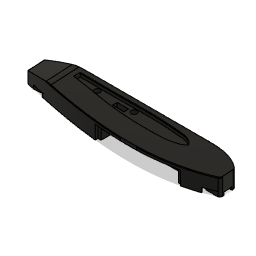
Rumpffräsung (Autodesk Fusion 360 archive; units mm, degrees)
design "Victor900_Rumpf_L"
Autodesk Fusion 360 part; units mm, degrees
(part 1 of 2)
sketch "Skizze1" plane through (0, 0, 0) normal (0, 1, 0) x (1, 0, 0)
  line L0 (-130, 18) -> (210, 18)
  line L1 (210, 18) -> (210, -52)
  line L2 (210, -52) -> (-130, -52)
  line L3 (-130, -52) -> (-130, 18)
  dimension "d132" = 70
  dimension "d133" = 130
  dimension "d134" = 18
  dimension "d135" = 340
  constraint horizontal L0
  constraint vertical L1
  constraint horizontal L2
  constraint vertical L3
  measures "d132" distance of L0.start L2.end
  measures "d133" distance of origin L3
  measures "d134" distance of origin L0
  measures "d135" distance of L1.end L2.end
extrude "Extrusion1" add sketch "Skizze1" along normal blind 5 and the other way blind 25
sketch "Skizze2" plane through (0, 5, 0) normal (0, 1, 0) x (-1, 0, 0)
  line L0 (130, 52) -> (-210, 52)
  line L1 (-210, 52) -> (-210, -18)
  line L2 (-210, -18) -> (130, -18)
  line L3 (130, -18) -> (130, 52)
  spline S0 degree 5 poles (-210, 26) (-205.2364, 28.1616) (-195.5185, 32.2752) (-180.3701, 37.8161) (-159.0102, 43.925) (-130.2557, 49.2993) (-99.3092, 52.2606) (-66.073, 52.7014) (-30.619, 50.7009) (6.8654, 46.4652) (46.175, 40.2203) (78.9412, 33.773) (104.2065, 28.1772) (121.3518, 24.1145) (130, 22) knots 0 0 0 0 0 0 0.1 0.2 0.3 0.4 0.5 0.6 0.7 0.8 0.9 1 1 1 1 1 1
  spline S1 degree 5 poles (-210, 2) (-208.6315, 0.7563) (-205.7512, -1.6794) (-201.0016, -5.1784) (-193.7504, -9.5129) (-182.4072, -14.1098) (-170.3603, -16.7165) (-158.8134, -17.7665) (-149.8205, -18) (-145, -18) knots 0 0 0 0 0 0 0.2 0.4 0.6 0.8 1 1 1 1 1 1
  line L4 (-155, -18) -> (-135, -18)
  spline S2 degree 5 poles (130, -8) (127.9223, -8.6218) (123.6828, -9.8397) (117.0718, -11.5892) (107.7186, -13.7564) (94.6903, -16.0549) (82.5244, -17.3582) (71.9269, -17.8833) (64.1023, -18) (60, -18) knots 0 0 0 0 0 0 0.2 0.4 0.6 0.8 1 1 1 1 1 1
  line L5 (70, -18) -> (50, -18)
  line L6 (-210, 26) -> (-207.3088, -18)
  point P0 (-90, 52)
  dimension "d140" = 120
  dimension "d143" = 20
  dimension "d145" = 24
  dimension "d146" = 65
  dimension "d147" = 30
  dimension "d148" = 20
  dimension "d149" = 70
  dimension "d161" = 3.5
  dimension "d351" = 20
  dimension "d352" = 10
  constraint coincident L1 S0.start
  constraint coincident L0 P0
  constraint coincident L3 S0.end
  constraint coincident L1 S1.start
  constraint coincident L2 S1.end
  constraint midpoint S1.end L4
  constraint collinear L2 L4
  constraint coincident L3 S2.start
  constraint coincident L2 S2.end
  constraint midpoint S2.end L5
  constraint collinear L2 L5
  constraint coincident L2 L6.end
  measures "d140" distance of L1 P0
  measures "d143" distance of L4.start L4.end
  measures "d145" distance of S0.start S1.start
  measures "d146" distance of L1 S1.end
  measures "d147" distance of S0.end S2.start
  measures "d148" distance of L5.start L5.end
  measures "d149" distance of L3 S2.end
  measures "d161" angle of L1 L6
  measures "d351" distance of L1.end S1.start
  measures "d352" distance of L2.end S2.start
extrude "Extrusion2" cut sketch "Skizze2" against normal blind 40 contours L0 L3 S0 | L0 L1 S0 | L2 L3 S2 L5 | L1 S1 L6 | L1 L2 S1 L6 | L2 S1 L4 L6
sketch "Skizze3" plane through (0, 5, 0) normal (0, 1, 0) x (-1, 0, 0)
  spline S0 degree 5 poles (-208.4486, 0.6348) (-207.3338, -0.3155) (-204.6874, -2.4507) (-200.1926, -5.6566) (-193.2477, -9.7166) (-182.4072, -14.1098) (-170.3603, -16.7165) (-158.8134, -17.7665) (-149.8205, -18) (-145, -18) knots 0.044317 0.044317 0.044317 0.044317 0.044317 0.044317 0.2 0.4 0.6 0.8 1 1 1 1 1 1
  line L0 (-145, -18) -> (60, -18)
  spline S1 degree 5 poles (60, -18) (64.1023, -18) (71.9269, -17.8833) (82.5244, -17.3582) (94.6903, -16.0549) (107.7186, -13.7564) (117.0718, -11.5892) (123.6828, -9.8397) (127.9223, -8.6218) (130, -8) knots -1 -1 -1 -1 -1 -1 -0.8 -0.6 -0.4 -0.2 0 0 0 0 0 0
  line L1 (130, -8) -> (130, 22)
  spline S2 degree 5 poles (130, 22) (121.3518, 24.1145) (104.2065, 28.1772) (78.9412, 33.773) (46.175, 40.2203) (7.677, 46.3363) (-21.5732, 49.6777) (-42.4683, 51.2272) (-55.7647, 51.8176) (-61.9632, 52) knots -1 -1 -1 -1 -1 -1 -0.9 -0.8 -0.7 -0.6 -0.510324 -0.510324 -0.510324 -0.510324 -0.510324 -0.510324
  line L2 (-61.9632, 52) -> (-90, 52)
  line L3 (130, -8) -> (128.4074, 22.3885)
  line L4 (129.2037, 7.1943) -> (-168.7369, -8.4202) construction
  line L5 (-210, 26) -> (-208.4486, 0.6348)
  spline S3 degree 5 poles (-90, 52) (-91.7641, 51.9445) (-100.03, 51.6408) (-114.4799, 50.739) (-134.4555, 48.5144) (-159.0102, 43.925) (-180.3701, 37.8161) (-195.5185, 32.2752) (-205.2364, 28.1616) (-210, 26) knots -0.426972 -0.426972 -0.426972 -0.426972 -0.426972 -0.426972 -0.4 -0.3 -0.2 -0.1 0 0 0 0 0 0
  dimension "d154" = 3
  constraint coincident S1.end L1.start
  constraint coincident S2 L3.end
  constraint midpoint L3 L4.start
  constraint perpendicular L3 L4
  measures "d154" angle of L1 L3
extrude "Extrusion3" cut sketch "Skizze3" against normal blind 47 contours L1 S2 L3
ref_plane "Arbeitsebene1" through (40, 0, 17) normal (0, 1, 0) x (0, 0, 1)
sketch "Skizze4" plane through (27.5, 0, 3) normal (0, 1, 0) x (1, 0, 0)
  line L0 (-97.7103, 1.804) -> (-97.7103, 13.2279)
  spline S0 degree 5 poles (-97.7103, 13.2279) (-96.5236, 13.2308) (-93.9185, 13.2352) (-90.1894, 13.2341) (-85.749, 13.2174) (-80.8951, 13.1754) (-76.1251, 13.1176) (-71.0655, 13.0567) (-65.2033, 13.0032) (-58.2308, 12.9668) (-50.1822, 12.9539) (-41.3331, 12.9683) (-32.096, 13.0103) (-22.9177, 13.0771) (-14.1775, 13.1622) (-6.0829, 13.255) (1.4285, 13.3413) (8.5923, 13.4029) (15.7306, 13.4191) (23.1596, 13.3663) (31.1056, 13.2202) (39.6032, 12.953) (48.4974, 12.5463) (57.5071, 11.9937) (66.2205, 11.3341) (74.2213, 10.6113) (80.9203, 10.0066) (86.1005, 9.5493) (90.5962, 8.6856) (95.1878, 6.918) (99.7425, 4.2895) (102.7176, 1.9586) (104.0892, 0.3889) (104.5631, -0.5029) (104.6892, -0.8472) knots -0.850912 -0.850912 -0.850912 -0.850912 -0.850912 -0.850912 -0.828571 -0.8 -0.771429 -0.742857 -0.714286 -0.685714 -0.657143 -0.628571 -0.6 -0.571429 -0.542857 -0.514286 -0.485714 -0.457143 -0.428571 -0.4 -0.371429 -0.342857 -0.314286 -0.285714 -0.257143 -0.228571 -0.2 -0.171429 -0.142857 -0.114286 -0.085714 -0.057143 -0.028571 -0.009156 -0.009156 -0.009156 -0.009156 -0.009156 -0.009156
  spline S1 degree 3 poles (104.6892, -0.8472) (104.7839, -1.1058) (104.8386, -1.3762) (104.8386, -1.6214) (104.8386, -2.5356) (104.213, -3.5125) (103.0553, -4.509) (101.9361, -5.4725) (100.3269, -6.4501) (98.4058, -7.3673) (96.5485, -8.2542) (94.4054, -9.0815) (92.1316, -9.8016) (89.9332, -10.4978) (87.6126, -11.0945) (85.2619, -11.5861) (82.9892, -12.0615) (80.6879, -12.4397) (78.4044, -12.7378) (74.0423, -13.3073) (69.7631, -13.5879) (65.6078, -13.7673) (61.7251, -13.9348) (57.9384, -14.0206) (54.1004, -14.0826) (50.5143, -14.1405) (46.8739, -14.1725) (43.0512, -14.1644) (39.4793, -14.1567) (35.7425, -14.1108) (31.8309, -14.012) (28.176, -13.9197) (24.3726, -13.7815) (20.5153, -13.6027) (16.9111, -13.4356) (13.2643, -13.2337) (9.6785, -13.0077) (6.328, -12.7966) (3.0333, -12.5647) (-0.1432, -12.3189) (-3.1112, -12.0892) (-5.9746, -11.8475) (-8.7301, -11.5932) (-11.3049, -11.3556) (-13.7868, -11.1067) (-16.2144, -10.8408) (-18.4827, -10.5922) (-20.7048, -10.3285) (-22.929, -10.0433) (-27.0353, -9.5168) (-31.1588, -8.9145) (-35.5916, -8.2103) (-39.4497, -7.5975) (-43.5436, -6.9077) (-47.9372, -6.155) (-51.7612, -5.4998) (-55.8084, -4.7979) (-60.059, -4.0715) (-63.7585, -3.4393) (-67.6104, -2.7889) (-71.5828, -2.1377) (-78.4142, -1.0179) (-85.5958, 0.1013) (-92.9594, 1.1447) (-94.5348, 1.368) (-96.1189, 1.5879) (-97.7103, 1.804) knots 0 0 0 0 0.00882694 0.00882694 0.00882694 0.04173953 0.04173953 0.04173953 0.07355923 0.07355923 0.07355923 0.10432234 0.10432234 0.10432234 0.13406394 0.13406394 0.13406394 0.16281794 0.16281794 0.16281794 0.21774546 0.21774546 0.21774546 0.26906918 0.26906918 0.26906918 0.31702555 0.31702555 0.31702555 0.3618355 0.3618355 0.3618355 0.40370548 0.40370548 0.40370548 0.44282836 0.44282836 0.44282836 0.47938439 0.47938439 0.47938439 0.51354198 0.51354198 0.51354198 0.54545849 0.54545849 0.54545849 0.57528096 0.57528096 0.57528096 0.63034008 0.63034008 0.63034008 0.67826152 0.67826152 0.67826152 0.7199706 0.7199706 0.7199706 0.75627265 0.75627265 0.75627265 0.81870207 0.81870207 0.81870207 0.8320585 0.8320585 0.8320585 0.8320585
extrude "Extrusion4" cut sketch "Skizze4" along normal blind 30
fillet "Abrundung2" radius 5 2 edges at (210, -10, 26) (208.4486, -10, 0.6348)
sketch "Skizze6" plane through (0, -25, 0) normal (0, -1, 0) x (1, 0, 0)
  spline S0 degree 3 poles (208.5813, 2.8044) (208.5416, 2.1546) (208.3753, 1.5187) (207.9292, 0.5965) (207.7295, 0.2796) (207.2633, -0.3037) (206.9983, -0.5683) (206.7063, -0.8009) knots 0 0 0 0 0.195322 0.195322 0.307328 0.307328 0.419333 0.419333 0.419333 0.419333
  line L0 (208.5813, 2.8044) -> (209.7883, 22.5389)
  line L1 (90, 52) -> (61.9632, 52)
  spline S1 degree 3 poles (61.9632, 52) (31.8484, 51.1138) (0.7584, 47.5087) (-61.8469, 37.484) (-95.8238, 30.3193) (-128.4074, 22.3885) knots 0 0 0 0 9.038353 9.038353 19.164916 19.164916 19.164916 19.164916
  line L2 (-128.4074, 22.3885) -> (-130, -8)
  spline S2 degree 3 poles (-130, -8) (-122.2961, -10.3057) (-112.1158, -12.9457) (-88.0124, -17.0435) (-75.2267, -18) (-60, -18) knots 0 0 0 0 2.412467 2.412467 5.223942 5.223942 5.223942 5.223942
  line L3 (-60, -18) -> (145, -18)
  spline S3 degree 3 poles (145, -18) (162.314, -18) (175.3428, -16.1927) (195.2364, -8.9464) (201.9978, -4.5522) (206.7063, -0.8009) knots 0 0 0 0 5.194191 5.194191 9.349234 9.349234 9.349234 9.349234
  line L4 (209.6335, 20.0079) -> (199.6522, 20.6184)
  line L5 (199.6522, 20.6184) -> (198.7547, 5.9458)
  line L6 (198.7547, 5.9458) -> (208.7361, 5.3354)
  line L7 (209.1848, 12.6716) -> (199.2035, 13.2821) construction
  line L8 (199.6522, 20.6184) -> (199.7987, 23.0139)
  line L9 (199.7987, 23.0139) -> (187.8211, 23.7465)
  line L10 (187.8211, 23.7465) -> (186.6306, 4.2829)
  line L11 (186.6306, 4.2829) -> (198.6082, 3.5503)
  line L12 (198.6082, 3.5503) -> (198.7547, 5.9458)
  line L13 (187.2258, 14.0147) -> (199.2035, 13.2821) construction
  spline S4 degree 3 poles (206.8011, 27.4252) (207.3976, 27.1643) (207.9375, 26.7894) (208.8431, 25.8537) (209.2002, 25.3019) (209.5778, 24.3557) (209.676, 24.0003) (209.7927, 23.2742) (209.8108, 22.9059) (209.7883, 22.5389) knots 0 0 0 0 0.195322 0.195322 0.390644 0.390644 0.500949 0.500949 0.611253 0.611253 0.611253 0.611253
  spline S5 degree 3 poles (206.8011, 27.4252) (190.0948, 34.7315) (172.6088, 40.2679) (133.4369, 48.918) (111.8704, 51.3122) (90, 52) knots 0.350203 0.350203 0.350203 0.350203 5.82041 5.82041 12.339895 12.339895 12.339895 12.339895
  dimension "d164" = 14.7
  dimension "d165" = 10
  dimension "d166" = 19.5
  dimension "d168" = 12
  constraint coincident L0 L4.start
  constraint perpendicular L0 L4
  constraint perpendicular L4 L5
  constraint coincident L0 L6.end
  constraint perpendicular L0 L6
  constraint midpoint L0 L7.start
  constraint midpoint L5 L7.end
  constraint perpendicular L5 L7
  constraint perpendicular L4 L8
  constraint perpendicular L8 L9
  constraint perpendicular L10 L11
  constraint perpendicular L6 L12
  constraint perpendicular L9 L10
  constraint midpoint L10 L13.start
  constraint perpendicular L10 L13
  measures "d164" distance of L4 L6
  measures "d165" distance of L0 L5
  measures "d166" distance of L9 L11
  measures "d168" distance of L5 L10
extrude "Extrusion5" cut sketch "Skizze6" against normal blind 10 contours L5 L8 L9 L10 L11 L12
extrude "Extrusion6" cut sketch "Skizze6" against normal blind 7 contours L0 L4 L5 L6
sketch "Skizze7" plane through (0, -25, 0) normal (0, -1, 0) x (1, 0, 0)
  line L0 (198.7547, 5.9458) -> (198.6082, 3.5503)
  line L1 (198.6082, 3.5503) -> (186.6306, 4.2829)
  line L2 (186.6306, 4.2829) -> (187.8211, 23.7465)
  line L3 (187.8211, 23.7465) -> (199.7987, 23.0139)
  line L4 (199.7987, 23.0139) -> (199.6522, 20.6184)
  line L5 (209.6335, 20.0079) -> (209.7883, 22.5389)
  line L6 (90, 52) -> (61.9632, 52)
  spline S0 degree 3 poles (61.9632, 52) (31.8484, 51.1138) (0.7584, 47.5087) (-61.8469, 37.484) (-95.8238, 30.3193) (-128.4074, 22.3885) knots 0 0 0 0 9.038353 9.038353 19.164916 19.164916 19.164916 19.164916
  line L7 (-128.4074, 22.3885) -> (-130, -8)
  spline S1 degree 3 poles (-130, -8) (-122.2961, -10.3057) (-112.1158, -12.9457) (-88.0124, -17.0435) (-75.2267, -18) (-60, -18) knots 0 0 0 0 2.412467 2.412467 5.223942 5.223942 5.223942 5.223942
  line L8 (-60, -18) -> (145, -18)
  spline S2 degree 3 poles (145, -18) (162.314, -18) (175.3428, -16.1927) (195.2364, -8.9464) (201.9978, -4.5522) (206.7063, -0.8009) knots 0 0 0 0 5.194191 5.194191 9.349234 9.349234 9.349234 9.349234
  spline S3 degree 3 poles (208.5813, 2.8044) (208.5416, 2.1546) (208.3753, 1.5187) (207.9292, 0.5965) (207.7295, 0.2796) (207.2633, -0.3037) (206.9983, -0.5683) (206.7063, -0.8009) knots 0 0 0 0 0.195322 0.195322 0.307328 0.307328 0.419333 0.419333 0.419333 0.419333
  line L9 (208.5813, 2.8044) -> (208.7361, 5.3354)
  line L10 (-118, -11.2728) -> (-116.6759, -1.3609)
  line L11 (-116.6759, -1.3609) -> (-67.1161, -7.9816)
  line L12 (-67.1161, -7.9816) -> (-68.4403, -17.8935)
  line L13 (208.7361, 5.3354) -> (198.7547, 5.9458)
  line L14 (199.6522, 20.6184) -> (209.6335, 20.0079)
  spline S4 degree 3 poles (206.8011, 27.4252) (207.3976, 27.1643) (207.9375, 26.7894) (208.8431, 25.8537) (209.2002, 25.3019) (209.5778, 24.3557) (209.676, 24.0003) (209.7927, 23.2742) (209.8108, 22.9059) (209.7883, 22.5389) knots 0 0 0 0 0.195322 0.195322 0.390644 0.390644 0.500949 0.500949 0.611253 0.611253 0.611253 0.611253
  spline S5 degree 3 poles (206.8011, 27.4252) (190.0948, 34.7315) (172.6088, 40.2679) (133.4369, 48.918) (111.8704, 51.3122) (90, 52) knots 0.350203 0.350203 0.350203 0.350203 5.82041 5.82041 12.339895 12.339895 12.339895 12.339895
  dimension "d175" = 50
  dimension "d176" = 12
  dimension "d177" = 10
  constraint coincident S1 L10.start
  constraint coincident S1 L12.end
  constraint perpendicular L11 L12
  constraint perpendicular L10 L11
  constraint equal L10 L12
  measures "d175" distance of L10 L12
  measures "d176" horizontal distance of L7.end L10.start
  measures "d177" distance of L10.start L11
extrude "Extrusion7" cut sketch "Skizze7" against normal blind 12.5 contours S1 L10 L11 L12
sketch "Skizze9" plane through (0, 0, 0) normal (0, 1, 0) x (-1, 0, 0)
  line L0 (70.2103, -10.2279) -> (70.2103, 1.196)
  line L1 (-20, 4) -> (0, 4)
  line L2 (0, 4) -> (0, -4)
  line L3 (0, -4) -> (-20, -4)
  line L4 (-20, -4) -> (-20, 4)
  line L5 (-20, 4) -> (0, -4) construction
  line L6 (0, 4) -> (-20, -4) construction
  spline S0 degree 5 poles (70.2103, -10.2279) (69.0236, -10.2308) (66.4185, -10.2352) (62.6894, -10.2341) (58.249, -10.2174) (53.3951, -10.1754) (48.6251, -10.1176) (43.5655, -10.0567) (37.7033, -10.0032) (30.7308, -9.9668) (22.6822, -9.9539) (13.8331, -9.9683) (4.596, -10.0103) (-4.5823, -10.0771) (-13.3225, -10.1622) (-21.4171, -10.255) (-28.9285, -10.3413) (-36.0923, -10.4029) (-43.2306, -10.4191) (-50.6596, -10.3663) (-58.6056, -10.2202) (-67.1032, -9.953) (-75.9974, -9.5463) (-85.0071, -8.9937) (-93.7205, -8.3341) (-101.7213, -7.6113) (-108.4203, -7.0066) (-113.6005, -6.5493) (-118.0962, -5.6856) (-122.6878, -3.918) (-127.2425, -1.2895) (-130.2176, 1.0414) (-131.5892, 2.6111) (-132.0631, 3.5029) (-132.1892, 3.8472) knots -0.850912 -0.850912 -0.850912 -0.850912 -0.850912 -0.850912 -0.828571 -0.8 -0.771429 -0.742857 -0.714286 -0.685714 -0.657143 -0.628571 -0.6 -0.571429 -0.542857 -0.514286 -0.485714 -0.457143 -0.428571 -0.4 -0.371429 -0.342857 -0.314286 -0.285714 -0.257143 -0.228571 -0.2 -0.171429 -0.142857 -0.114286 -0.085714 -0.057143 -0.028571 -0.009156 -0.009156 -0.009156 -0.009156 -0.009156 -0.009156
  spline S1 degree 3 poles (-132.1892, 3.8472) (-132.2839, 4.1058) (-132.3386, 4.3762) (-132.3386, 4.6214) (-132.3386, 5.5356) (-131.713, 6.5125) (-130.5553, 7.509) (-129.4361, 8.4725) (-127.8269, 9.4501) (-125.9058, 10.3673) (-124.0485, 11.2542) (-121.9054, 12.0815) (-119.6316, 12.8016) (-117.4332, 13.4978) (-115.1126, 14.0945) (-112.7619, 14.5861) (-110.4892, 15.0615) (-108.1879, 15.4397) (-105.9044, 15.7378) (-101.5423, 16.3073) (-97.2631, 16.5879) (-93.1078, 16.7673) (-89.2251, 16.9348) (-85.4384, 17.0206) (-81.6004, 17.0826) (-78.0143, 17.1405) (-74.3739, 17.1725) (-70.5512, 17.1644) (-66.9793, 17.1567) (-63.2425, 17.1108) (-59.3309, 17.012) (-55.676, 16.9197) (-51.8726, 16.7815) (-48.0153, 16.6027) (-44.4111, 16.4356) (-40.7643, 16.2337) (-37.1785, 16.0077) (-33.828, 15.7966) (-30.5333, 15.5647) (-27.3568, 15.3189) (-24.3888, 15.0892) (-21.5254, 14.8475) (-18.7699, 14.5932) (-16.1951, 14.3556) (-13.7132, 14.1067) (-11.2856, 13.8408) (-9.0173, 13.5922) (-6.7952, 13.3285) (-4.571, 13.0433) (-0.4647, 12.5168) (3.6588, 11.9145) (8.0916, 11.2103) (11.9497, 10.5975) (16.0436, 9.9077) (20.4372, 9.155) (24.2612, 8.4998) (28.3084, 7.7979) (32.559, 7.0715) (36.2585, 6.4393) (40.1104, 5.7889) (44.0828, 5.1377) (50.9142, 4.0179) (58.0958, 2.8987) (65.4594, 1.8553) (67.0348, 1.632) (68.6189, 1.4121) (70.2103, 1.196) knots 0 0 0 0 0.00882694 0.00882694 0.00882694 0.04173953 0.04173953 0.04173953 0.07355923 0.07355923 0.07355923 0.10432234 0.10432234 0.10432234 0.13406394 0.13406394 0.13406394 0.16281794 0.16281794 0.16281794 0.21774546 0.21774546 0.21774546 0.26906918 0.26906918 0.26906918 0.31702555 0.31702555 0.31702555 0.3618355 0.3618355 0.3618355 0.40370548 0.40370548 0.40370548 0.44282836 0.44282836 0.44282836 0.47938439 0.47938439 0.47938439 0.51354198 0.51354198 0.51354198 0.54545849 0.54545849 0.54545849 0.57528096 0.57528096 0.57528096 0.63034008 0.63034008 0.63034008 0.67826152 0.67826152 0.67826152 0.7199706 0.7199706 0.7199706 0.75627265 0.75627265 0.75627265 0.81870207 0.81870207 0.81870207 0.8320585 0.8320585 0.8320585 0.8320585
  point P0 (-10, 0)
  dimension "d213" = 8
  dimension "d214" = 20
  dimension "d653" = 10
  constraint horizontal L1
  constraint perpendicular L1 L2
  constraint parallel L1 L3
  constraint parallel L2 L4
  constraint coincident L5 P0
  constraint coincident L6 P0
  constraint horizontal origin P0
  measures "d213" distance of L1.end L2.end
  measures "d214" distance of L1.start L1.end
  measures "d653" distance of origin P0
extrude "Extrusion9" cut sketch "Skizze9" against normal blind 43 contours L1 L2 L3 L4
sketch "Skizze10" plane through (0, -25, 0) normal (0, -1, 0) x (1, 0, 0)
  line L0 (-118, -11.2728) -> (-116.6759, -1.3609)
  line L1 (-116.6759, -1.3609) -> (-67.1161, -7.9816)
  line L2 (-67.1161, -7.9816) -> (-68.4403, -17.8935)
  spline S0 degree 3 poles (-68.4403, -17.8935) (-65.7031, -17.9654) (-62.8957, -18) (-60, -18) knots 4.689279 4.689279 4.689279 4.689279 5.223942 5.223942 5.223942 5.223942
  line L3 (-60, -18) -> (145, -18)
  spline S1 degree 3 poles (145, -18) (162.314, -18) (175.3428, -16.1927) (195.2364, -8.9464) (201.9978, -4.5522) (206.7063, -0.8009) knots 0 0 0 0 5.194191 5.194191 9.349234 9.349234 9.349234 9.349234
  spline S2 degree 3 poles (208.5813, 2.8044) (208.5416, 2.1546) (208.3753, 1.5187) (207.9292, 0.5965) (207.7295, 0.2796) (207.2633, -0.3037) (206.9983, -0.5683) (206.7063, -0.8009) knots 0 0 0 0 0.195322 0.195322 0.307328 0.307328 0.419333 0.419333 0.419333 0.419333
  line L4 (208.5813, 2.8044) -> (208.7361, 5.3354)
  line L5 (198.7547, 5.9458) -> (198.6082, 3.5503)
  line L6 (198.6082, 3.5503) -> (186.6306, 4.2829)
  line L7 (186.6306, 4.2829) -> (187.8211, 23.7465)
  line L8 (187.8211, 23.7465) -> (199.7987, 23.0139)
  line L9 (199.7987, 23.0139) -> (199.6522, 20.6184)
  line L10 (90, 52) -> (61.9632, 52)
  spline S3 degree 3 poles (61.9632, 52) (31.8484, 51.1138) (0.7584, 47.5087) (-61.8469, 37.484) (-95.8238, 30.3193) (-128.4074, 22.3885) knots 0 0 0 0 9.038353 9.038353 19.164916 19.164916 19.164916 19.164916
  line L11 (-128.4074, 22.3885) -> (-130, -8)
  spline S4 degree 3 poles (-130, -8) (-126.471, -9.0562) (-122.4223, -10.1826) (-118, -11.2728) knots 0 0 0 0 1.105113 1.105113 1.105113 1.105113
  line L12 (186.6306, 4.2829) -> (151.6306, 4.2829)
  line L13 (151.6306, 4.2829) -> (151.6306, 24.2829)
  line L14 (151.6306, 24.2829) -> (186.6306, 24.2829)
  line L15 (186.6306, 24.2829) -> (186.6306, 4.2829)
  line L16 (186.6306, 24.2829) -> (187.8211, 23.7465)
  line L17 (0, -4) -> (0, 4)
  line L18 (0, 4) -> (20, 4)
  line L19 (20, 4) -> (20, -4)
  line L20 (20, -4) -> (0, -4)
  line L21 (208.7361, 5.3354) -> (198.7547, 5.9458)
  line L22 (199.6522, 20.6184) -> (209.6335, 20.0079)
  line L23 (209.6335, 20.0079) -> (209.7883, 22.5389)
  spline S5 degree 3 poles (206.8011, 27.4252) (207.3976, 27.1643) (207.9375, 26.7894) (208.8431, 25.8537) (209.2002, 25.3019) (209.5778, 24.3557) (209.676, 24.0003) (209.7927, 23.2742) (209.8108, 22.9059) (209.7883, 22.5389) knots 0 0 0 0 0.195322 0.195322 0.390644 0.390644 0.500949 0.500949 0.611253 0.611253 0.611253 0.611253
  spline S6 degree 3 poles (206.8011, 27.4252) (190.0948, 34.7315) (172.6088, 40.2679) (133.4369, 48.918) (111.8704, 51.3122) (90, 52) knots 0.350203 0.350203 0.350203 0.350203 5.82041 5.82041 12.339895 12.339895 12.339895 12.339895
  dimension "d195" = 35
  dimension "d196" = 20
  constraint horizontal L12
  constraint vertical L13
  constraint horizontal L14
  constraint vertical L15
  constraint coincident L6.end L7.start
  constraint coincident L7.end L8.start
  measures "d195" distance of L6.end L12.end
  measures "d196" distance of L6.end L14.end
extrude "Extrusion10" cut sketch "Skizze10" against normal blind 20 contours L7 L15 L16 | L12 L13 L14 L15
sketch "Skizze11" plane through (0, -25, 0) normal (0, -1, 0) x (1, 0, 0)
  line L0 (186.6306, 4.2829) -> (151.6306, 4.2829)
  line L1 (151.6306, 4.2829) -> (151.6306, 24.2829)
  line L2 (151.6306, 24.2829) -> (186.6306, 24.2829)
  line L3 (186.6306, 24.2829) -> (187.8211, 23.7465)
  line L4 (187.8211, 23.7465) -> (199.7987, 23.0139)
  line L5 (199.7987, 23.0139) -> (199.6522, 20.6184)
  line L6 (209.6335, 20.0079) -> (209.7883, 22.5389)
  line L7 (90, 52) -> (61.9632, 52)
  spline S0 degree 3 poles (61.9632, 52) (31.8484, 51.1138) (0.7584, 47.5087) (-61.8469, 37.484) (-95.8238, 30.3193) (-128.4074, 22.3885) knots 0 0 0 0 9.038353 9.038353 19.164916 19.164916 19.164916 19.164916
  line L8 (-128.4074, 22.3885) -> (-130, -8)
  spline S1 degree 3 poles (-130, -8) (-126.471, -9.0562) (-122.4223, -10.1826) (-118, -11.2728) knots 0 0 0 0 1.105113 1.105113 1.105113 1.105113
  line L9 (-118, -11.2728) -> (-116.6759, -1.3609)
  line L10 (-116.6759, -1.3609) -> (-67.1161, -7.9816)
  line L11 (-67.1161, -7.9816) -> (-68.4403, -17.8935)
  spline S2 degree 3 poles (-68.4403, -17.8935) (-65.7031, -17.9654) (-62.8957, -18) (-60, -18) knots 4.689279 4.689279 4.689279 4.689279 5.223942 5.223942 5.223942 5.223942
  line L12 (-60, -18) -> (145, -18)
  spline S3 degree 3 poles (145, -18) (162.314, -18) (175.3428, -16.1927) (195.2364, -8.9464) (201.9978, -4.5522) (206.7063, -0.8009) knots 0 0 0 0 5.194191 5.194191 9.349234 9.349234 9.349234 9.349234
  spline S4 degree 3 poles (208.5813, 2.8044) (208.5416, 2.1546) (208.3753, 1.5187) (207.9292, 0.5965) (207.7295, 0.2796) (207.2633, -0.3037) (206.9983, -0.5683) (206.7063, -0.8009) knots 0 0 0 0 0.195322 0.195322 0.307328 0.307328 0.419333 0.419333 0.419333 0.419333
  line L13 (208.5813, 2.8044) -> (208.7361, 5.3354)
  line L14 (198.6082, 3.5503) -> (186.6306, 4.2829)
  line L15 (206.8011, 34.4252) -> (186.8011, 34.4252)
  line L16 (186.8011, 34.4252) -> (186.8011, 27.4252)
  line L17 (186.8011, 27.4252) -> (206.8011, 27.4252)
  line L18 (206.8011, 27.4252) -> (206.8011, 34.4252)
  spline S5 degree 5 poles (186.8011, 34.4252) (185.3367, 34.4252) (182.5917, 34.349) (179.0243, 34.0062) (175.1755, 33.1206) (171.0793, 31.292) (167.7239, 29.1134) (164.856, 26.9379) (162.7398, 25.2136) (161.6306, 24.2829) knots 0 0 0 0 0 0 0.2 0.4 0.6 0.8 1 1 1 1 1 1
  line L19 (189.3011, 34.4252) -> (184.3011, 34.4252)
  line L20 (163.5457, 25.8899) -> (159.7155, 22.6759)
  line L21 (0, -4) -> (0, 4)
  line L22 (0, 4) -> (20, 4)
  line L23 (20, 4) -> (20, -4)
  line L24 (20, -4) -> (0, -4)
  line L25 (199.6522, 20.6184) -> (209.6335, 20.0079)
  line L26 (208.7361, 5.3354) -> (198.7547, 5.9458)
  line L27 (198.7547, 5.9458) -> (198.6082, 3.5503)
  spline S6 degree 3 poles (206.8011, 27.4252) (207.3976, 27.1643) (207.9375, 26.7894) (208.8431, 25.8537) (209.2002, 25.3019) (209.5778, 24.3557) (209.676, 24.0003) (209.7927, 23.2742) (209.8108, 22.9059) (209.7883, 22.5389) knots 0 0 0 0 0.195322 0.195322 0.390644 0.390644 0.500949 0.500949 0.611253 0.611253 0.611253 0.611253
  spline S7 degree 3 poles (206.8011, 27.4252) (190.0948, 34.7315) (172.6088, 40.2679) (133.4369, 48.918) (111.8704, 51.3122) (90, 52) knots 0.350203 0.350203 0.350203 0.350203 5.82041 5.82041 12.339895 12.339895 12.339895 12.339895
  spline S8 degree 5 poles (186.8011, 27.4252) (186.7106, 27.4252) (186.4576, 27.3757) (185.8619, 27.1533) (184.7264, 26.6117) (183.1509, 25.7374) (182.1411, 25.0505) (181.7235, 24.6221) (181.6306, 24.3875) (181.6306, 24.2829) knots 0 0 0 0 0 0 0.2 0.4 0.6 0.8 1 1 1 1 1 1
  line L28 (181.6306, 24.7829) -> (181.6306, 23.7829)
  line L29 (187.3011, 27.4252) -> (186.3011, 27.4252)
  dimension "d199" = 7
  dimension "d201" = 20
  dimension "d202" = 40
  dimension "d203" = 5
  dimension "d534" = 10
  dimension "d535" = 1
  dimension "d536" = 20
  constraint horizontal L15
  constraint vertical L16
  constraint horizontal L17
  constraint vertical L18
  constraint midpoint L15.end L19
  constraint collinear L15 L19
  constraint midpoint S5.end L20
  constraint equal L19 L20
  constraint coincident L17.end L18.start
  constraint coincident L2 S5.end
  constraint coincident L2 S8.end
  constraint midpoint S8.end L28
  constraint vertical L28
  constraint midpoint L16.end L29
  constraint collinear L17 L29
  constraint equal L28 L29
  measures "d199" distance of L15 L17
  measures "d201" distance of L15.start L15.end
  measures "d202" angle of L2 L20
  measures "d203" distance of L19.start L19.end
  measures "d534" distance of L1 S5.end
  measures "d535" distance of L29.start L29.end
  measures "d536" distance of S5.end S8.end
extrude "Extrusion11" cut sketch "Skizze11" against normal blind 10 contours L2 L16 S5 S8 | L15 L16 L17 L19 S7 L29 | L15 L18 L19 S7
fillet "Abrundung4" radius 0.5 1 edges at (189.0696, -20, 34.4252)
sketch "Skizze12" plane through (0, -25, 0) normal (0, -1, 0) x (1, 0, 0)
  line L0 (90, 52) -> (61.9632, 52)
  spline S0 degree 3 poles (61.9632, 52) (31.8484, 51.1138) (0.7584, 47.5087) (-61.8469, 37.484) (-95.8238, 30.3193) (-128.4074, 22.3885) knots 0 0 0 0 9.038353 9.038353 19.164916 19.164916 19.164916 19.164916
  line L1 (-128.4074, 22.3885) -> (-130, -8)
  spline S1 degree 3 poles (-130, -8) (-126.471, -9.0562) (-122.4223, -10.1826) (-118, -11.2728) knots 0 0 0 0 1.105113 1.105113 1.105113 1.105113
  line L2 (-118, -11.2728) -> (-116.6759, -1.3609)
  line L3 (-116.6759, -1.3609) -> (-67.1161, -7.9816)
  line L4 (-67.1161, -7.9816) -> (-68.4403, -17.8935)
  spline S2 degree 3 poles (-68.4403, -17.8935) (-65.7031, -17.9654) (-62.8957, -18) (-60, -18) knots 4.689279 4.689279 4.689279 4.689279 5.223942 5.223942 5.223942 5.223942
  line L5 (-60, -18) -> (145, -18)
  spline S3 degree 3 poles (145, -18) (162.314, -18) (175.3428, -16.1927) (195.2364, -8.9464) (201.9978, -4.5522) (206.7063, -0.8009) knots 0 0 0 0 5.194191 5.194191 9.349234 9.349234 9.349234 9.349234
  spline S4 degree 3 poles (208.5813, 2.8044) (208.5416, 2.1546) (208.3753, 1.5187) (207.9292, 0.5965) (207.7295, 0.2796) (207.2633, -0.3037) (206.9983, -0.5683) (206.7063, -0.8009) knots 0 0 0 0 0.195322 0.195322 0.307328 0.307328 0.419333 0.419333 0.419333 0.419333
  line L6 (198.6082, 3.5503) -> (186.6306, 4.2829)
  line L7 (186.6306, 4.2829) -> (151.6306, 4.2829)
  line L8 (151.6306, 4.2829) -> (151.6306, 24.2829)
  line L9 (151.6306, 24.2829) -> (161.6306, 24.2829)
  spline S5 degree 5 poles (161.6306, 24.2829) (162.7398, 25.2136) (164.856, 26.9379) (167.7239, 29.1134) (171.0793, 31.292) (175.0993, 33.0866) (178.8457, 33.9647) (182.2619, 34.3162) (184.831, 34.409) (186.1282, 34.4219) knots -1 -1 -1 -1 -1 -1 -0.8 -0.6 -0.4 -0.2 -0.018597 -0.018597 -0.018597 -0.018597 -0.018597 -0.018597
  line L10 (0, -4) -> (0, 4)
  line L11 (0, 4) -> (20, 4)
  line L12 (20, 4) -> (20, -4)
  line L13 (20, -4) -> (0, -4)
  line L14 (0, 5) -> (-70, 5)
  line L15 (-70, 5) -> (-70, 20)
  line L16 (-70, 20) -> (0, 20)
  line L17 (0, 20) -> (0, 5)
  line L18 (0, 20) -> (20, 20)
  line L19 (20, 20) -> (20, 4)
  line L20 (20, 4) -> (0, 4)
  line L21 (0, 5) -> (0, 4)
  line L22 (208.7361, 5.3354) -> (198.7547, 5.9458)
  line L23 (208.5813, 2.8044) -> (208.7361, 5.3354)
  line L24 (198.7547, 5.9458) -> (198.6082, 3.5503)
  spline S6 degree 3 poles (186.2852, 35.3949) (175.963, 38.9282) (165.419, 41.8556) (133.4369, 48.918) (111.8704, 51.3122) (90, 52) knots 2.550857 2.550857 2.550857 2.550857 5.82041 5.82041 12.339895 12.339895 12.339895 12.339895
  spline S7 degree 3 poles (186.2852, 35.3949) (186.3468, 35.3738) (186.4037, 35.3409) (186.5017, 35.2551) (186.5418, 35.2031) (186.5999, 35.0865) (186.6172, 35.0231) (186.6267, 34.8932) (186.6187, 34.828) (186.5781, 34.7043) (186.546, 34.6469) (186.4615, 34.5479) (186.41, 34.5071) (186.3175, 34.4595) (186.2811, 34.4458) (186.2057, 34.4272) (186.1671, 34.4222) (186.1282, 34.4219) knots 0 0 0 0 0.019532 0.019532 0.039064 0.039064 0.058597 0.058597 0.078129 0.078129 0.097661 0.097661 0.117193 0.117193 0.128841 0.128841 0.140488 0.140488 0.140488 0.140488
  dimension "d216" = 70
  dimension "d217" = 15
  dimension "d666" = 9
  constraint horizontal L14
  constraint vertical L15
  constraint horizontal L16
  constraint horizontal L18
  constraint vertical L19
  constraint horizontal L20
  constraint coincident L11 L12.start
  constraint coincident L10.end L11.start
  constraint collinear L10 L21
  constraint collinear L17 L21
  constraint coincident L11.end L12.start
  measures "d216" distance of L14.start L14.end
  measures "d217" distance of L14.start L16.end
  measures "d666" distance of L13 L14
extrude "Extrusion12" cut sketch "Skizze12" against normal blind 20 contours L11 L17 L18 L19 L20 L21 | L14 L15 L16 L17
sketch "Skizze13" plane through (0, -25, 0) normal (0, -1, 0) x (1, 0, 0)
  line L0 (90, 52) -> (61.9632, 52)
  spline S0 degree 3 poles (61.9632, 52) (31.8484, 51.1138) (0.7584, 47.5087) (-61.8469, 37.484) (-95.8238, 30.3193) (-128.4074, 22.3885) knots 0 0 0 0 9.038353 9.038353 19.164916 19.164916 19.164916 19.164916
  line L1 (-128.4074, 22.3885) -> (-130, -8)
  spline S1 degree 3 poles (-130, -8) (-126.471, -9.0562) (-122.4223, -10.1826) (-118, -11.2728) knots 0 0 0 0 1.105113 1.105113 1.105113 1.105113
  line L2 (-118, -11.2728) -> (-116.6759, -1.3609)
  line L3 (-116.6759, -1.3609) -> (-67.1161, -7.9816)
  line L4 (-67.1161, -7.9816) -> (-68.4403, -17.8935)
  spline S2 degree 3 poles (-68.4403, -17.8935) (-65.7031, -17.9654) (-62.8957, -18) (-60, -18) knots 4.689279 4.689279 4.689279 4.689279 5.223942 5.223942 5.223942 5.223942
  line L5 (-60, -18) -> (145, -18)
  spline S3 degree 3 poles (145, -18) (162.314, -18) (175.3428, -16.1927) (195.2364, -8.9464) (201.9978, -4.5522) (206.7063, -0.8009) knots 0 0 0 0 5.194191 5.194191 9.349234 9.349234 9.349234 9.349234
  spline S4 degree 3 poles (208.5813, 2.8044) (208.5416, 2.1546) (208.3753, 1.5187) (207.9292, 0.5965) (207.7295, 0.2796) (207.2633, -0.3037) (206.9983, -0.5683) (206.7063, -0.8009) knots 0 0 0 0 0.195322 0.195322 0.307328 0.307328 0.419333 0.419333 0.419333 0.419333
  line L6 (198.6082, 3.5503) -> (186.6306, 4.2829)
  line L7 (186.6306, 4.2829) -> (151.6306, 4.2829)
  line L8 (151.6306, 4.2829) -> (151.6306, 24.2829)
  line L9 (151.6306, 24.2829) -> (161.6306, 24.2829)
  spline S5 degree 5 poles (161.6306, 24.2829) (162.7398, 25.2136) (164.856, 26.9379) (167.7239, 29.1134) (171.0793, 31.292) (175.0993, 33.0866) (178.8457, 33.9647) (182.2619, 34.3162) (184.831, 34.409) (186.1282, 34.4219) knots -1 -1 -1 -1 -1 -1 -0.8 -0.6 -0.4 -0.2 -0.018597 -0.018597 -0.018597 -0.018597 -0.018597 -0.018597
  line L10 (0, -4) -> (0, 5)
  line L11 (0, 5) -> (-70, 5)
  line L12 (-70, 5) -> (-70, 20)
  line L13 (-70, 20) -> (20, 20)
  line L14 (20, 20) -> (20, -4)
  line L15 (20, -4) -> (0, -4)
  line L16 (20, 52) -> (151.6306, 52)
  line L17 (151.6306, 52) -> (151.6306, 5)
  line L18 (151.6306, 5) -> (20, 5)
  line L19 (20, 5) -> (20, 52)
  line L20 (151.6306, 4.2829) -> (150.3886, 5)
  line L21 (208.7361, 5.3354) -> (198.7547, 5.9458)
  line L22 (208.5813, 2.8044) -> (208.7361, 5.3354)
  line L23 (198.7547, 5.9458) -> (198.6082, 3.5503)
  spline S6 degree 3 poles (186.2852, 35.3949) (175.963, 38.9282) (165.419, 41.8556) (133.4369, 48.918) (111.8704, 51.3122) (90, 52) knots 2.550857 2.550857 2.550857 2.550857 5.82041 5.82041 12.339895 12.339895 12.339895 12.339895
  spline S7 degree 3 poles (186.2852, 35.3949) (186.3468, 35.3738) (186.4037, 35.3409) (186.5017, 35.2551) (186.5418, 35.2031) (186.5999, 35.0865) (186.6172, 35.0231) (186.6267, 34.8932) (186.6187, 34.828) (186.5781, 34.7043) (186.546, 34.6469) (186.4615, 34.5479) (186.41, 34.5071) (186.3175, 34.4595) (186.2811, 34.4458) (186.2057, 34.4272) (186.1671, 34.4222) (186.1282, 34.4219) knots 0 0 0 0 0.019532 0.019532 0.039064 0.039064 0.058597 0.058597 0.078129 0.078129 0.097661 0.097661 0.117193 0.117193 0.128841 0.128841 0.140488 0.140488 0.140488 0.140488
  dimension "d229" = 30
  constraint horizontal L16
  constraint vertical L17
  constraint horizontal L18
  constraint vertical L19
  constraint collinear L0 L16
  constraint collinear L8 L17
  constraint coincident L7.end L8.start
  constraint coincident L18 L20.end
  constraint collinear L14 L19
  constraint collinear L11 L18
  measures "d229" angle of L18 L20
extrude "Extrusion14" cut sketch "Skizze13" against normal blind 20 contours L0 S0 L8 L14 L16 L17 L18 L19 S6 | L16 L17 S6 | S0 L16 L19
sketch "Skizze14" plane through (0, -25, 0) normal (0, -1, 0) x (1, 0, 0)
  line L0 (208.5813, 2.8044) -> (208.7361, 5.3354)
  line L1 (198.7547, 5.9458) -> (198.6082, 3.5503)
  spline S0 degree 5 poles (-70, 20) (-70.649, 20) (-71.8766, 20.059) (-73.5073, 20.3247) (-75.34, 21.0237) (-77.4768, 22.4066) (-79.8449, 24.1445) (-82.7026, 26.0217) (-85.7353, 27.5823) (-88.7356, 28.6279) (-91.7149, 29.2006) (-94.1422, 29.3883) (-96.036, 29.4467) (-97.3386, 29.4597) (-98, 29.4597) knots 0 0 0 0 0 0 0.1 0.2 0.3 0.4 0.5 0.6 0.7 0.8 0.9 1 1 1 1 1 1
  line L2 (-67, 20) -> (-73, 20)
  line L3 (-95.2026, 29.4597) -> (-100.7974, 29.4597)
  spline S1 degree 5 poles (-70, 11) (-71.1795, 11) (-73.2304, 11.0683) (-75.3791, 11.3749) (-76.9214, 12.2119) (-78.7301, 13.9682) (-82.4088, 16.3513) (-87.0611, 18.8953) (-91.6017, 21.1928) (-96.185, 23.0654) (-101.2284, 24.4154) (-106.2045, 25.0605) (-110.7485, 25.301) (-114.1821, 25.3544) (-116, 25.3544) knots 0 0 0 0 0 0 0.1 0.2 0.3 0.4 0.5 0.6 0.7 0.8 0.9 1 1 1 1 1 1
  line L4 (-111, 25.3544) -> (-121, 25.3544)
  line L5 (-64.6288, 11) -> (-75.3712, 11)
  line L6 (-79.4402, 23.9356) -> (-84.5598, 27.0644)
  line L7 (-79.4402, 14.4356) -> (-84.5598, 17.5644)
  line L8 (-116, 25.3544) -> (-98, 29.4597) construction
  line L9 (-70, 11) -> (-70, 20)
  line L10 (-116, 25.3544) -> (-98, 29.4597)
  line L11 (20, 20) -> (20, 49.205)
  spline S2 degree 3 poles (20, 49.205) (3.5548, 47.5578) (-12.8338, 45.3322) (-61.8469, 37.484) (-95.8238, 30.3193) (-128.4074, 22.3885) knots 4.160884 4.160884 4.160884 4.160884 9.038353 9.038353 19.164916 19.164916 19.164916 19.164916
  line L12 (-128.4074, 22.3885) -> (-130, -8)
  spline S3 degree 3 poles (-130, -8) (-126.471, -9.0562) (-122.4223, -10.1826) (-118, -11.2728) knots 0 0 0 0 1.105113 1.105113 1.105113 1.105113
  line L13 (-118, -11.2728) -> (-116.6759, -1.3609)
  line L14 (-116.6759, -1.3609) -> (-67.1161, -7.9816)
  line L15 (-67.1161, -7.9816) -> (-68.4403, -17.8935)
  spline S4 degree 3 poles (-68.4403, -17.8935) (-65.7031, -17.9654) (-62.8957, -18) (-60, -18) knots 4.689279 4.689279 4.689279 4.689279 5.223942 5.223942 5.223942 5.223942
  line L16 (-60, -18) -> (145, -18)
  spline S5 degree 3 poles (145, -18) (162.314, -18) (175.3428, -16.1927) (195.2364, -8.9464) (201.9978, -4.5522) (206.7063, -0.8009) knots 0 0 0 0 5.194191 5.194191 9.349234 9.349234 9.349234 9.349234
  spline S6 degree 3 poles (208.5813, 2.8044) (208.5416, 2.1546) (208.3753, 1.5187) (207.9292, 0.5965) (207.7295, 0.2796) (207.2633, -0.3037) (206.9983, -0.5683) (206.7063, -0.8009) knots 0 0 0 0 0.195322 0.195322 0.307328 0.307328 0.419333 0.419333 0.419333 0.419333
  line L17 (208.7361, 5.3354) -> (198.7547, 5.9458)
  line L18 (198.6082, 3.5503) -> (186.6306, 4.2829)
  line L19 (186.6306, 4.2829) -> (151.6306, 4.2829)
  line L20 (151.6306, 5) -> (20, 5)
  line L21 (20, 5) -> (20, -4)
  line L22 (20, -4) -> (0, -4)
  line L23 (0, -4) -> (0, 5)
  line L24 (0, 5) -> (-70, 5)
  line L25 (-70, 5) -> (-70, 20)
  line L26 (-70, 20) -> (20, 20)
  line L27 (151.6306, 4.2829) -> (151.6306, 5)
  line L28 (-70, 5) -> (-67.1161, -7.9816)
  line L29 (-81.6096, 15.7592) -> (-76.6175, -6.7123)
  point P0 (-82, 25.5)
  point P1 (-82, 16)
  dimension "d253" = 9
  dimension "d254" = 9.5
  dimension "d322" = 18
  dimension "d588" = 12
  dimension "d589" = 10
  dimension "d604" = 28
  dimension "d684" = 11
  dimension "d685" = 6
  dimension "d716" = 9
  constraint midpoint S0.start L2
  constraint midpoint S0.end L3
  constraint horizontal L3
  constraint midpoint S1.end L4
  constraint horizontal L4
  constraint midpoint S1.start L5
  constraint horizontal L5
  constraint midpoint P0 L6
  constraint midpoint P1 L7
  constraint parallel L6 L7
  constraint equal L6 L7
  constraint vertical P0 P1
  constraint vertical S0.start S1.start
  constraint coincident S1.end S2
  constraint coincident S0.end S2
  constraint coincident L2 S0.start
  constraint coincident L9 S0.start
  constraint coincident L2.end L6
  constraint equal L2 L6
  constraint coincident L24.end L25.start
  constraint coincident L14.end L15.start
  constraint coincident S1 L29.start
  constraint coincident L14 L29.end
  constraint parallel L28 L29
  measures "d253" distance of L2 L5
  measures "d254" distance of P0 P1
  measures "d322" distance of S0.end S1.end
  measures "d588" distance of P0 L9
  measures "d589" distance of L4.start L4.end
  measures "d604" distance of S0.end L9
  measures "d684" distance of P1 L24
  measures "d685" distance of L2.start L2.end
  measures "d716" distance of L28 L29
extrude "Extrusion15" cut sketch "Skizze14" against normal blind 8 contours S1 L14 L25 L28 L29 | S0 S1 L9 L10 L25 | L10 S2
extrude "Extrusion18" add 1 faces at (160.2695, 5, 8.6046) along direction (0, 1, 0) blind 2
sketch "Skizze15" plane through (0, -25, 0) normal (0, -1, 0) x (1, 0, 0)
  line L0 (350, 100) -> (-350, 100)
  line L1 (-350, 100) -> (-350, -100)
  line L2 (-350, -100) -> (350, -100)
  line L3 (350, -100) -> (350, 100)
  line L4 (350, 100) -> (-350, -100) construction
  line L5 (-350, 100) -> (350, -100) construction
  spline S0 degree 5 poles (-81.6096, 15.7592) (-81.8101, 15.884) (-82.7906, 16.487) (-84.7064, 17.6027) (-87.7297, 19.2336) (-91.6017, 21.1928) (-96.185, 23.0654) (-101.2284, 24.4154) (-106.2045, 25.0605) (-110.7485, 25.301) (-114.1821, 25.3544) (-116, 25.3544) knots 0.373627 0.373627 0.373627 0.373627 0.373627 0.373627 0.4 0.5 0.6 0.7 0.8 0.9 1 1 1 1 1 1
  spline S1 degree 3 poles (-116, 25.3544) (-120.155, 24.3795) (-124.2923, 23.3901) (-128.4074, 22.3885) knots 17.885992 17.885992 17.885992 17.885992 19.164916 19.164916 19.164916 19.164916
  line L6 (-128.4074, 22.3885) -> (-130, -8)
  spline S2 degree 3 poles (-130, -8) (-126.471, -9.0562) (-122.4223, -10.1826) (-118, -11.2728) knots 0 0 0 0 1.105113 1.105113 1.105113 1.105113
  line L7 (-118, -11.2728) -> (-116.6759, -1.3609)
  line L8 (-116.6759, -1.3609) -> (-76.6175, -6.7123)
  line L9 (-76.6175, -6.7123) -> (-81.6096, 15.7592)
  dimension "d495" = 200
  dimension "d496" = 700
  constraint horizontal L0
  constraint perpendicular L0 L1
  constraint parallel L0 L2
  constraint parallel L1 L3
  constraint coincident L4 origin
  constraint coincident L5 origin
  measures "d495" distance of L0.start L2.end
  measures "d496" distance of L0.start L0.end
extrude "Extrusion19" cut sketch "Skizze15" against normal blind 2 contours L0 L1 L2 L3 | S0 S1 L6 S2 L7 L8 L9
fillet "Abrundung14" radius 0.2 1 edges at (-98, -20, 29.4597)
sketch "Skizze17" plane through (0, -23, 0) normal (0, -1, 0) x (1, 0, 0)
  line L0 (10, 42.1329) -> (-70, 29.3498)
  line L1 (-70, 29.3498) -> (-70, 20)
  line L2 (10, 42.1329) -> (10, 20)
  spline S0 degree 3 poles (-96.2959, 29.8359) (-73.617, 34.8269) (-50.6209, 39.2985) (-12.3394, 45.3991) (3.8016, 47.5825) (20, 49.205) knots -15.877269 -15.877269 -15.877269 -15.877269 -8.967074 -8.967074 -4.161468 -4.161468 -4.161468 -4.161468
  line L3 (-70, 35.3498) -> (10, 48.1329) construction
  line L4 (-70, 20) -> (-70, 5)
  spline S1 degree 3 poles (-96.2575, 29.4406) (-96.2835, 29.4412) (-96.3092, 29.4469) (-96.3569, 29.4677) (-96.3785, 29.4827) (-96.4148, 29.5202) (-96.429, 29.5422) (-96.4483, 29.5906) (-96.4532, 29.6164) (-96.4527, 29.6685) (-96.4473, 29.6943) (-96.4271, 29.7423) (-96.4124, 29.7641) (-96.3805, 29.7957) (-96.3653, 29.8071) (-96.3321, 29.8251) (-96.3144, 29.8318) (-96.2959, 29.8359) knots 0 0 0 0 0.007813 0.007813 0.015626 0.015626 0.023439 0.023439 0.031252 0.031252 0.039064 0.039064 0.046877 0.046877 0.052542 0.052542 0.058207 0.058207 0.058207 0.058207
  spline S2 degree 3 poles (-70, 20) (-71.9866, 20) (-73.4142, 20.3317) (-75.9479, 21.3955) (-77.1136, 22.194) (-80.5065, 24.5643) (-83.1643, 26.4546) (-89.1611, 28.8236) (-91.9919, 29.3428) (-96.2575, 29.4406) knots -5.427911 -5.427911 -5.427911 -5.427911 -4.367525 -4.367525 -3.227892 -3.227892 -1.580801 -1.580801 -0.182146 -0.182146 -0.182146 -0.182146
  line L5 (-70, 20) -> (20, 20)
  line L6 (20, 20) -> (20, 49.205)
  spline S3 degree 3 poles (-96.2959, 29.8359) (-73.617, 34.8269) (-50.6209, 39.2985) (-12.3394, 45.3991) (3.8016, 47.5825) (20, 49.205) knots -15.877269 -15.877269 -15.877269 -15.877269 -8.967074 -8.967074 -4.161468 -4.161468 -4.161468 -4.161468
  dimension "d305" = 6
  dimension "d306" = 6
  dimension "d687" = 10
  constraint coincident S0 L3.start
  constraint coincident S0 L3.end
  constraint coincident L2 L3.end
  constraint coincident L1 L3.start
  constraint vertical L2
  constraint coincident L2.end L5
  constraint collinear L1 L4
  measures "d305" distance of L0.end L3.start
  measures "d306" distance of L0.start L3.end
  measures "d687" distance of L2 L6
extrude "Extrusion21" cut sketch "Skizze17" against normal up to surface (18 mm away) contours L0 L1 L2 L5
fillet "Abrundung15" radius 6 1 edges at (10, -14, 20)
ref_plane "Arbeitsebene2" through (-128.4074, -9, 22.3885) normal (0.052336, 0, 0.99863) x (0, -1, 0)
sketch "Skizze19" plane through (-123.6824, -9, 22.1409) normal (0.052336, 0, 0.99863) x (0, -1, 0)
  line L0 (-6, -4.7315) -> (-17, -4.7315)
  line L1 (-17, -4.7315) -> (-17, 45.2685)
  line L2 (-17, 45.2685) -> (-6, -4.7315)
  line L3 (-16, 332.8204) -> (-16, 331.1366)
  line L4 (-16, 331.1366) -> (-16, 270.415)
  line L5 (-16, 270.415) -> (-16, 65.696)
  line L6 (-16, 65.696) -> (-16, -4.7315)
  line L7 (-16, -4.7315) -> (-16, 183.8285)
  line L8 (-16, 183.8285) -> (-16, 211.8269)
  line L9 (-16, 332.9929) -> (-16, 332.8204)
  line L10 (-16, 54.495) -> (-16, 55.0929)
  line L11 (-16, 211.8269) -> (-16, 329.7541)
  line L12 (-16, 329.7541) -> (-16, 332.9931)
  line L13 (-16, 256.5887) -> (-16, 54.495)
  line L14 (-16, 55.0929) -> (-16, 256.4784)
  dimension "d356" = 1
  dimension "d357" = 50
  dimension "d360" = 11
  constraint horizontal L0
  constraint perpendicular L0 L1
  constraint coincident L0 L6.end
  measures "d356" distance of L1 L6
  measures "d357" distance of L0.end L1.end
  measures "d360" distance of L0.start L0.end
extrude "Extrusion22" cut sketch "Skizze19" along normal through all and the other way through all
fillet "Abrundung16" radius 50 2 edges at (-83.6474, 7, 7.9461) (-83.6474, 7, 7.9461)
sketch "Skizze20" plane through (0, -23, 0) normal (0, -1, 0) x (1, 0, 0)
  spline S0 degree 3 poles (-96.2959, 29.8359) (-73.617, 34.8269) (-50.6209, 39.2985) (-12.3394, 45.3991) (3.8016, 47.5825) (20, 49.205) knots -15.877269 -15.877269 -15.877269 -15.877269 -8.967074 -8.967074 -4.161468 -4.161468 -4.161468 -4.161468
  line L0 (20.5724, 50.0976) -> (14.5724, 50.0976)
  line L1 (14.5724, 50.0976) -> (14.5724, 46.0976)
  line L2 (14.5724, 46.0976) -> (20.5724, 46.0976)
  line L3 (20.5724, 46.0976) -> (20.5724, 50.0976)
  line L4 (151.6306, 44.8836) -> (157.6306, 44.8836)
  line L5 (157.6306, 44.8836) -> (157.6306, 40.8836)
  line L6 (157.6306, 40.8836) -> (151.6306, 40.8836)
  line L7 (151.6306, 40.8836) -> (151.6306, 44.8836)
  spline S1 degree 5 poles (90, 52) (91.7641, 51.9445) (100.03, 51.6408) (114.4799, 50.739) (134.4555, 48.5144) (158.2419, 44.0686) (178.9415, 38.2222) (193.4896, 33.0097) (202.6297, 29.2495) (206.8011, 27.4252) knots -0.426972 -0.426972 -0.426972 -0.426972 -0.426972 -0.426972 -0.4 -0.3 -0.2 -0.1 -0.013359 -0.013359 -0.013359 -0.013359 -0.013359 -0.013359
  line L8 (61.9632, 52) -> (90, 52)
  line L9 (14.5724, 43.7809) -> (14.5724, 50.0976)
  line L10 (14.5724, 43.7809) -> (164.5724, 43.7809)
  line L11 (164.5724, 43.7809) -> (164.5724, 53.7809)
  line L12 (164.5724, 53.7809) -> (14.5724, 53.7809)
  line L13 (14.5724, 53.7809) -> (14.5724, 43.7809)
  line L14 (15.4029, 43.7809) -> (151.6306, 40.8836)
  arc A0 (10, 26) -> (16, 20) centre (16, 26) ccw
  line L15 (16, 20) -> (20, 20)
  line L16 (20, 20) -> (20, 49.205)
  spline S2 degree 3 poles (-96.2575, 29.4406) (-96.2835, 29.4412) (-96.3092, 29.4469) (-96.3569, 29.4677) (-96.3785, 29.4827) (-96.4148, 29.5202) (-96.429, 29.5422) (-96.4483, 29.5906) (-96.4532, 29.6164) (-96.4527, 29.6685) (-96.4473, 29.6943) (-96.4271, 29.7423) (-96.4124, 29.7641) (-96.3805, 29.7957) (-96.3653, 29.8071) (-96.3321, 29.8251) (-96.3144, 29.8318) (-96.2959, 29.8359) knots 0 0 0 0 0.007813 0.007813 0.015626 0.015626 0.023439 0.023439 0.031252 0.031252 0.039064 0.039064 0.046877 0.046877 0.052542 0.052542 0.058207 0.058207 0.058207 0.058207
  spline S3 degree 3 poles (-70, 20) (-71.9866, 20) (-73.4142, 20.3317) (-75.9479, 21.3955) (-77.1136, 22.194) (-80.5065, 24.5643) (-83.1643, 26.4546) (-89.1611, 28.8236) (-91.9919, 29.3428) (-96.2575, 29.4406) knots -5.427911 -5.427911 -5.427911 -5.427911 -4.367525 -4.367525 -3.227892 -3.227892 -1.580801 -1.580801 -0.182146 -0.182146 -0.182146 -0.182146
  line L17 (-70, 20) -> (-70, 29.3498)
  line L18 (-70, 29.3498) -> (10, 42.1329)
  line L19 (10, 42.1329) -> (10, 26)
  point P0 (20, 49.205)
  point P1 (151.6306, 44.8836)
  dimension "d559" = 6
  dimension "d560" = 4
  dimension "d562" = 150
  dimension "d563" = 10
  constraint horizontal L0
  constraint vertical L1
  constraint horizontal L2
  constraint vertical L3
  constraint horizontal L4
  constraint vertical L5
  constraint horizontal L6
  constraint vertical L7
  constraint coincident P1 L4.start
  constraint equal L2 L6
  constraint equal L1 L5
  constraint perpendicular L0 L9
  constraint horizontal L10
  constraint vertical L11
  constraint horizontal L12
  constraint vertical L13
  constraint coincident L10 L14.start
  measures "d559" distance of L0.start L0.end
  measures "d560" distance of L0.start L2.end
  measures "d562" distance of L9.start L10.end
  measures "d563" distance of L9.start L12.end
extrude "Extrusion23" cut sketch "Skizze20" against normal blind 24 contours S0 L0 L1 L2 L3 L9 L13 L16 | S0 L1 L2 L9 L13 L16 | L0 L2 L3 L4 L5 L7 L10 L11 L12 L13 L16 | L2 L9 L10 L13 L16 | L7 L10 L14 L16 | L5 L6 L7 S1 L10 | L7 S1 L10 | L4 L5 S1 L10 | L5 S1 L10
extrude "Extrusion26" cut 1 faces at (163.2973, -14.3333, 4.2829) along direction (0, 0, 1) up to surface (0.7171 mm away)
fillet "Abrundung18" radius 5 2 edges at (10, -14, 42.1329) (151.6306, -14, 5)